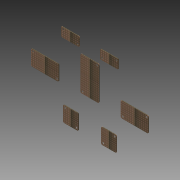
# Autodesk Inventor part: Bottom Plate Veroboard
Saved by Autodesk Inventor 2015 (Build 190159000, 159)
## iProperties
Created: 2016-02-13
Part Number: Bottom Plate Veroboard
Material: Veroboard
Document SubType Name: Modeling
Designer: James
Density: 1 g/cm^3
Appearance: Generic
Author: James
Autodesk Inventor part; units mm, degrees
ref_plane "YZ Plane" through (0, 0, 0) normal (1, 0, 0) x (0, 1, 0)
ref_plane "XZ Plane" through (0, 0, 0) normal (0, 1, 0) x (-1, 0, 0)
ref_plane "XY Plane" through (0, 0, 0) normal (0, 0, 1) x (1, 0, 0)
sketch "Sketch1" plane through (0, 0, 0) normal (0, 1, 0) x (-1, 0, 0)
  line L0 (-38.2, -31.3) -> (-38.2, -52.3)
  arc A0 (-40.2, -54.3) -> (-38.2, -52.3) centre (-40.2, -52.3) ccw
  line L1 (-40.2, -54.3) -> (-81.2, -54.3)
  line L2 (-83.2, -52.3) -> (-83.2, -31.3)
  line L3 (-81.2, -29.3) -> (-40.2, -29.3)
  arc A1 (-38.2, -31.3) -> (-40.2, -29.3) centre (-40.2, -31.3) ccw
  arc A2 (-81.2, -29.3) -> (-83.2, -31.3) centre (-81.2, -31.3) ccw
  circle A3 centre (-41.4, -51.1) radius 1.6
  circle A4 centre (-80, -32.5) radius 1.6
  line L4 (61.8, -31.3) -> (61.8, -52.3)
  arc A5 (61.8, -52.3) -> (63.8, -54.3) centre (63.8, -52.3) ccw
  line L5 (63.8, -54.3) -> (104.8, -54.3)
  line L6 (106.8, -52.3) -> (106.8, -31.3)
  arc A6 (104.8, -54.3) -> (106.8, -52.3) centre (104.8, -52.3) ccw
  line L7 (104.8, -29.3) -> (63.8, -29.3)
  arc A7 (63.8, -29.3) -> (61.8, -31.3) centre (63.8, -31.3) ccw
  arc A8 (106.8, -31.3) -> (104.8, -29.3) centre (104.8, -31.3) ccw
  circle A9 centre (65, -51.1) radius 1.6
  circle A10 centre (103.6, -32.5) radius 1.6
  line L8 (-8.55, -107.3) -> (-29.55, -107.3)
  arc A11 (-31.55, -105.3) -> (-29.55, -107.3) centre (-29.55, -105.3) ccw
  line L9 (-31.55, -105.3) -> (-31.55, -84.3)
  arc A12 (-29.55, -82.3) -> (-31.55, -84.3) centre (-29.55, -84.3) ccw
  line L10 (-29.55, -82.3) -> (-8.55, -82.3)
  arc A13 (-6.55, -84.3) -> (-8.55, -82.3) centre (-8.55, -84.3) ccw
  line L11 (-6.55, -84.3) -> (-6.55, -105.3)
  arc A14 (-8.55, -107.3) -> (-6.55, -105.3) centre (-8.55, -105.3) ccw
  circle A15 centre (-28.35, -85.5) radius 1.6
  circle A16 centre (-9.75, -104.1) radius 1.6
  line L12 (32.15, -107.3) -> (53.15, -107.3)
  arc A17 (53.15, -107.3) -> (55.15, -105.3) centre (53.15, -105.3) ccw
  line L13 (55.15, -105.3) -> (55.15, -84.3)
  arc A18 (55.15, -84.3) -> (53.15, -82.3) centre (53.15, -84.3) ccw
  line L14 (53.15, -82.3) -> (32.15, -82.3)
  arc A19 (32.15, -82.3) -> (30.15, -84.3) centre (32.15, -84.3) ccw
  line L15 (30.15, -84.3) -> (30.15, -105.3)
  arc A20 (30.15, -105.3) -> (32.15, -107.3) centre (32.15, -105.3) ccw
  circle A21 centre (51.95, -85.5) radius 1.6
  circle A22 centre (33.35, -104.1) radius 1.6
  line L16 (26.8, 1.2) -> (26.8, -49.8)
  arc A23 (24.8, -51.8) -> (26.8, -49.8) centre (24.8, -49.8) ccw
  line L17 (24.8, -51.8) -> (-1.2, -51.8)
  line L18 (-3.2, -49.8) -> (-3.2, 1.2)
  arc A24 (-3.2, -49.8) -> (-1.2, -51.8) centre (-1.2, -49.8) ccw
  line L19 (24.8, 3.2) -> (-1.2, 3.2)
  arc A25 (-1.2, 3.2) -> (-3.2, 1.2) centre (-1.2, 1.2) ccw
  arc A26 (26.8, 1.2) -> (24.8, 3.2) centre (24.8, 1.2) ccw
  line L20 (-6.7451, 25.9447) -> (-32.7451, 25.9447)
  arc A27 (-4.7451, 23.9447) -> (-6.7451, 25.9447) centre (-6.7451, 23.9447) ccw
  arc A28 (-32.7451, 25.9447) -> (-34.7451, 23.9447) centre (-32.7451, 23.9447) ccw
  line L21 (-34.7451, 23.9447) -> (-34.7451, 12.9447)
  line L22 (-4.7451, 23.9447) -> (-4.7451, 12.9447)
  arc A29 (-6.7451, 10.9447) -> (-4.7451, 12.9447) centre (-6.7451, 12.9447) ccw
  circle A30 centre (-31.5451, 22.7447) radius 1.6
  circle A31 centre (-7.9451, 14.1447) radius 1.6
  line L23 (-32.7451, 10.9447) -> (-6.7451, 10.9447)
  arc A32 (-34.7451, 12.9447) -> (-32.7451, 10.9447) centre (-32.7451, 12.9447) ccw
  line L24 (30.3451, 25.9447) -> (56.3451, 25.9447)
  arc A33 (30.3451, 25.9447) -> (28.3451, 23.9447) centre (30.3451, 23.9447) ccw
  arc A34 (58.3451, 23.9447) -> (56.3451, 25.9447) centre (56.3451, 23.9447) ccw
  line L25 (58.3451, 23.9447) -> (58.3451, 12.9447)
  line L26 (28.3451, 23.9447) -> (28.3451, 12.9447)
  arc A35 (28.3451, 12.9447) -> (30.3451, 10.9447) centre (30.3451, 12.9447) ccw
  circle A36 centre (55.1451, 22.7447) radius 1.6
  circle A37 centre (31.5451, 14.1447) radius 1.6
  line L27 (56.3451, 10.9447) -> (30.3451, 10.9447)
  arc A38 (56.3451, 10.9447) -> (58.3451, 12.9447) centre (56.3451, 12.9447) ccw
  circle A39 centre (23.6, -48.6) radius 1.6
  circle A40 centre (0, 0) radius 1.6
  arc A41 (-83.2, -52.3) -> (-81.2, -54.3) centre (-81.2, -52.3) ccw
  constraints: 56 end point, 56 point on circle, 42 centre point
extrude "Extrusion1" add sketch "Sketch1" along normal blind 1
body "Solid1"
